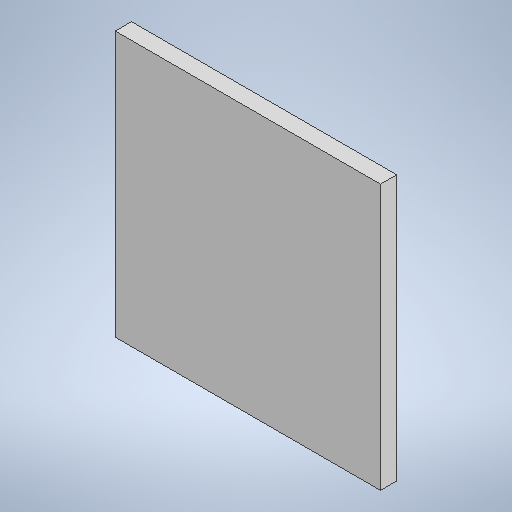
# Autodesk Inventor part: air layer
Saved by Autodesk Inventor 2025.1 (Build 291241020, 241B)
## iProperties
Created: 2024-10-29
Part Number: air layer
Material: Generic
Document SubType Name: Modeling
Designer: jjk
Density: 1 g/cm^3
Appearance: Default
Author: jjk
Autodesk Inventor part; units mm, degrees
ref_plane "YZ Plane" through (0, 0, 0) normal (1, 0, 0) x (0, 1, 0)
ref_plane "XZ Plane" through (0, 0, 0) normal (0, 1, 0) x (-1, 0, 0)
ref_plane "XY Plane" through (0, 0, 0) normal (0, 0, 1) x (1, 0, 0)
sketch "Sketch1" plane through (0, 0, 0) normal (0, 0, 1) x (1, 0, 0)
  line L0 (0, 0) -> (152.4, 0)
  line L1 (152.4, 0) -> (152.4, 152.4)
  line L2 (0, 152.4) -> (0, 0)
  line L3 (152.4, 152.4) -> (88.9, 152.4)
  line L4 (63.5, 152.4) -> (0, 152.4)
  line L5 (63.5, 0) -> (88.9, 0)
  line L6 (63.5, 152.4) -> (88.9, 152.4)
  line L7 (0, 152.4) -> (0, 0)
  line L8 (152.4, 0) -> (0, 0)
  constraints: 18 end point, 3 parallel, 2 horizontal, 2 perpendicular, 1 collinear, 1 point on line, 1 vertical
extrude "Extrusion1" add sketch "Sketch1" along normal blind 9.3218
body "Solid1"
